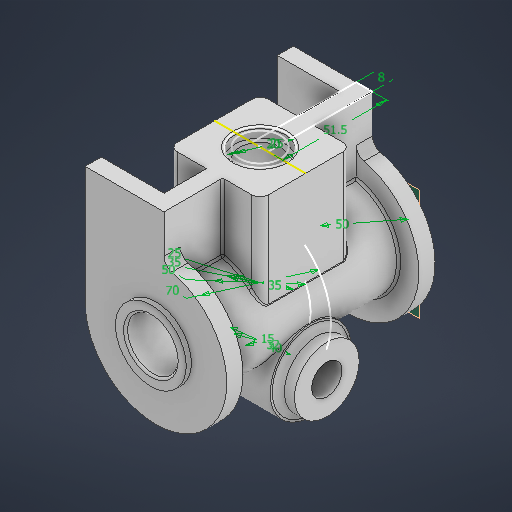
# Autodesk Inventor part: Day02_Task05
Saved by Autodesk Inventor 2026.3 (Build 303398000, 398)
## iProperties
Created: 2026-08-05
Part Number: Day02_Task05
Material: 일반
Document SubType Name: Modeling
Designer: hojin
Density: 1 g/cm^3
Appearance: 기본값
Author: hojin
Autodesk Inventor part; units mm, degrees
ref_plane "YZ Plane" through (0, 0, 0) normal (1, 0, 0) x (0, 1, 0)
ref_plane "XZ Plane" through (0, 0, 0) normal (0, 1, 0) x (-1, 0, 0)
ref_plane "XY Plane" through (0, 0, 0) normal (0, 0, 1) x (1, 0, 0)
sketch "스케치2" plane through (0, 0, 0) normal (0, 1, 0) x (-1, 0, 0)
  line L0 (22.5, 0) -> (-22.5, 0)
  line L1 (-22.5, 0) -> (-22.5, -22.5)
  line L2 (-22.5, -22.5) -> (22.5, -22.5)
  line L3 (22.5, -22.5) -> (22.5, 0)
  point P0 (0, 0)
  point P1 (0, 0)
  dimension "d2" = 45
  dimension "d3" = 22.5
  constraints: 8 end point, 2 parallel, 1 coincident, 1 horizontal, 1 midpoint, 1 perpendicular
  measures "d2" distance of L2.end L1.end
  measures "d3" distance of L1.end L0.end
extrude "돌출1" add sketch "스케치2" along normal blind 58
sketch "스케치3" plane through (0, 0, 0) normal (0, 0, 1) x (1, 0, 0)
  circle A0 centre (0, 0) radius 12.5
  circle A1 centre (0, 0) radius 17.5
  circle A2 centre (0, 0) radius 25
  circle A3 centre (0, 0) radius 35
  line L0 (22.5, 0) -> (-22.5, 0) projected
  dimension "d6" = 25
  dimension "d7" = 35
  dimension "d8" = 50
  dimension "d9" = 70
  constraints: 4 centre point, 3 concentric, 1 coincident, 1 midpoint
  measures "d6" diameter of A0
  measures "d7" diameter of A1
  measures "d8" diameter of A2
  measures "d9" diameter of A3
extrude "돌출2" add sketch "스케치3" against normal blind 54 contours L0 A1 A0 | A0 L0 A1
extrude "돌출3" add sketch "스케치3" against normal blind 51.5 contours A2
ref_plane "작업 평면1" through (0, 0, -51.5) normal (0, 0, -1) x (-1, 0, 0)
sketch "스케치4" plane through (0, 0, -51.5) normal (0, 0, -1) x (-1, 0, 0)
  circle A0 centre (0, 0) radius 35
  dimension "d15" = 70
  constraints: 1 centre point, 1 coincident
  measures "d15" diameter of A0
sketch "스케치5" plane through (0, 0, -51.5) normal (0, 0, -1) x (-1, 0, 0)
  circle A0 centre (0, 0) radius 25
  dimension "d16" = 50
  constraints: 1 centre point, 1 coincident
  measures "d16" diameter of A0
extrude "돌출4" add sketch "스케치4" against normal blind 8
extrude "돌출5" cut sketch "스케치3" against normal through all contours L0 A0 | A0 L0
sketch "스케치7" plane through (0, 58, 0) normal (0, 1, 0) x (1, 0, 0)
  line L0 (-4, 0) -> (4, 0)
  line L1 (4, 0) -> (4, 51.5)
  line L2 (4, 51.5) -> (-4, 51.5)
  line L3 (-4, 51.5) -> (-4, 0)
  line L4 (-22.5, 0) -> (22.5, 0) projected
  point P0 (0, 0)
  point P1 (0, 0)
  dimension "d21" = 8
  dimension "d22" = 51.5
  constraints: 8 end point, 2 midpoint, 2 parallel, 1 horizontal, 1 perpendicular
  measures "d21" distance of L2.end L1.end
  measures "d22" distance of L0.end L1.end
extrude "돌출6" add sketch "스케치7" against normal blind 30
extrude "돌출7" add sketch "스케치7" against normal blind 40
sketch "스케치8" plane through (0, 0, -51.5) normal (0, 0, -1) x (-1, 0, 0)
  line L0 (-4, 58) -> (35, 58)
  line L1 (35, 58) -> (35, 0)
  line L2 (35, 0) -> (-4, 0)
  line L3 (-4, 0) -> (-4, 58)
  arc A0 (-4, 34.7707) -> (4, 34.7707) centre (0, 0) ccw projected
  line L4 (-4, 58) -> (4, 58) projected
  point P0 (0, 58)
  dimension "d27" = 39
  dimension "d28" = 58
  constraints: 8 end point, 2 parallel, 1 horizontal, 1 midpoint, 1 perpendicular, 1 point on line, 1 tangent
  measures "d27" distance of L1.end L2.end
  measures "d28" distance of L0.end L1.end
extrude "돌출8" add sketch "스케치8" against normal blind 8 contours L0 L1 L2 L3
extrude "돌출9" cut sketch "스케치3" against normal through all contours L0 A0 | A0 L0
fillet "모깎기1" radius 1 1 edges at (-12.5, 0, -54)
fillet "모깎기2" radius 5 1 edges at (4, 34.7707, -47.5)
fillet "모깎기3" radius 4 2 edges at (-22.5, 34.4486, -22.5) (22.5, 34.4486, -22.5)
fillet "모깎기4" radius 1 10 edges at (11.9171, 21.9768, -22.5) (22.5, 10.8972, -9.25) (21.1633, 13.3084, -21.4844) (4, 41.339, -22.5) (4, 24.6779, -33) (-21.1633, 13.3084, -21.4844) (-11.9171, 21.9768, -22.5) (-22.5, 10.8972, -9.25) (-4, 24.6779, -33) (0, -25, -43.5)
mirror "미러1" about plane through (-22.5, 0, 0) normal (0, 0, 1)
sketch "스케치10" plane through (0, 58, 0) normal (0, 1, 0) x (1, 0, 0)
  circle A0 centre (0, 0) radius 12.5
  circle A1 centre (0, 0) radius 10
  dimension "d37" = 25
  dimension "d38" = 20
  constraints: 2 centre point, 1 coincident, 1 concentric
  measures "d37" diameter of A0
  measures "d38" diameter of A1
extrude "돌출10" cut sketch "스케치10" against normal up to next contours A1
extrude "돌출11" cut sketch "스케치10" against normal blind 5
fillet "모깎기5" radius 1 1 edges at (-12.5, 58, 0)
sketch "스케치11" plane through (0, 0, 0) normal (1, 0, 0) x (0, 1, 0)
  circle A0 centre (0, 0) radius 17.5
  circle A1 centre (-25, 0) radius 7.5
  circle A2 centre (-25, 0) radius 16
  circle A3 centre (-25, 0) radius 20
  point P0 (-13.505, 11.1295)
  point P1 (-13.505, -11.1295)
  point P2 (-17.5, 0)
  dimension "d44" = 35
  dimension "d45" = 15
  dimension "d46" = 32
  dimension "d47" = 40
  constraints: 4 centre point, 2 concentric, 1 coincident, 1 horizontal alignment, 1 tangent
  measures "d44" diameter of A0
  measures "d45" diameter of A1
  measures "d46" diameter of A2
  measures "d47" diameter of A3
extrude "돌출12" add sketch "스케치11" along normal mid plane 50 contours A0 A2 picked at (-19.7306, 11.971)
extrude "돌출13" add sketch "스케치11" along normal mid plane 66 contours A0 A2 picked at (-19.7306, 11.971)
extrude "돌출14" add sketch "스케치11" along normal mid plane 50 contours A3 A0 A2 | A0 A2 A3 | A2 A0 | A1 | A0 A2
extrude "돌출15" add sketch "스케치11" along normal mid plane 66 contours A2 A0 | A0 A2
extrude "돌출16" cut sketch "스케치11" along normal through all both and the other way through all contours A1
fillet "모깎기6" radius 3 6 edges at (-25, -41, 0) (-25, -10.169, -6.0033) (-25, -10.169, 6.0033) (25, -41, 0) (25, -10.169, -6.0033) (25, -10.169, 6.0033)
fillet "모깎기7" radius 1 1 edges at (-33, -32.5, 0)
extrude "돌출17" cut sketch "스케치3" along normal through all contours L0 A0 | A0 L0
extrude "돌출18" cut sketch "스케치3" along normal mid plane 10 contours L0 A0 | A0 L0
extrude "돌출19" cut sketch "스케치3" along normal through all both and the other way through all contours L0 A0 | A0 L0
